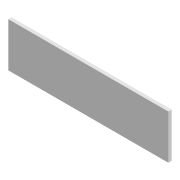
# Autodesk Inventor part: 00_Baseplate_Simmo_side4_v2
Saved by Autodesk Inventor 2022 (Build 260153000, 153)
## iProperties
Created: 2022-08-09
Part Number: 00_Baseplate_Simmo_side4_v2
Material: Generic
Document SubType Name: Modeling
Designer: wanghaoran
Density: 1 g/cm^3
Appearance: Default
Author: wanghaoran
Autodesk Inventor part; units mm, degrees
ref_plane "YZ Plane" through (0, 0, 0) normal (1, 0, 0) x (0, 1, 0)
ref_plane "XZ Plane" through (0, 0, 0) normal (0, 1, 0) x (-1, 0, 0)
ref_plane "XY Plane" through (0, 0, 0) normal (0, 0, 1) x (1, 0, 0)
sketch "Sketch1" plane through (0, 0, 0) normal (0, 0, 1) x (1, 0, 0)
  line L0 (-10, 0) -> (-10, 6) projected
  line L1 (275.4242, 0) -> (275.4242, 6) projected
  line L2 (275.4242, 6) -> (-10, 6)
  line L3 (-10, 6) -> (-10, -73)
  line L4 (-10, -73) -> (275.4242, -73)
  line L5 (275.4242, -73) -> (275.4242, 6)
  point P0 (0, 0)
  dimension "d0" = 79
  constraints: 8 end point, 2 parallel, 1 horizontal, 1 perpendicular
  measures "d0" distance of L3.end L2.end
extrude "Extrusion1" add sketch "Sketch1" along normal blind 6
body "Solid1"
